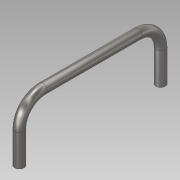
# Autodesk Inventor part: AGARRADERA
Saved by Autodesk Inventor 2019 (Build 230136000, 136)
## iProperties
Created: 2020-04-10
Part Number: AGARRADERA
Material: Acero inoxidable
Document SubType Name: Modeling
Designer: Luis Pujol
Density: 8 g/cm^3
Appearance: Semipulido
Author: Luis Pujol
Autodesk Inventor part; units mm, degrees
ref_plane "YZ Plane" through (0, 0, 0) normal (1, 0, 0) x (0, 1, 0)
ref_plane "XZ Plane" through (0, 0, 0) normal (0, 1, 0) x (-1, 0, 0)
ref_plane "XY Plane" through (0, 0, 0) normal (0, 0, 1) x (1, 0, 0)
sketch "Boceto1" plane through (0, 0, 0) normal (1, 0, 0) x (0, 1, 0)
  line L0 (0, 45.315) -> (20, 45.315)
  line L1 (35, 30.315) -> (35, -29.685)
  line L2 (20, -44.685) -> (0, -44.685)
  arc A0 (35, 30.315) -> (20, 45.315) centre (20, 30.315) ccw
  arc A1 (20, -44.685) -> (35, -29.685) centre (20, -29.685) ccw
  point P0 (0, 0)
  point P1 (35, 45.315)
  point P2 (35, -44.685)
  dimension "d0" = 35
  dimension "d1" = 90
  dimension "d2" = 15
  constraints: 6 end point, 4 point on circle, 4 point on line, 4 tangent, 2 centre point, 1 equal radius, 1 horizontal, 1 perpendicular
  measures "d0" distance of point (35, -44.685) L2.end
  measures "d1" distance of point (35, 45.315) point (35, -44.685)
  measures "d2" radius of A0
sketch "Boceto2" plane through (0, 0, 0) normal (0, 1, 0) x (-1, 0, 0)
  circle A0 centre (0, 45) radius 3
  point P0 (0, 0)
  dimension "d3" = 6
  constraints: 1 centre point
  measures "d3" diameter of A0
sweep "Barrido1" add profiles "Boceto2" path "Boceto1"
